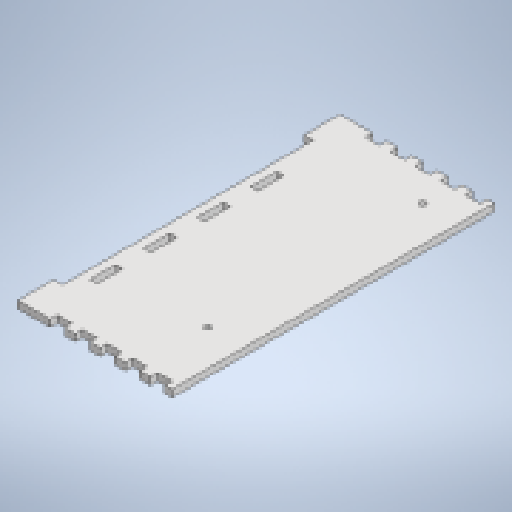
# Autodesk Inventor part: side
Saved by Autodesk Inventor 2025.3 (Build 293356000, 356)
## iProperties
Created: 2025-12-08
Part Number: side
Material: Generic
Document SubType Name: Modeling
Designer: hazem
Density: 1 g/cm^3
Appearance: Default
Author: hazem
Autodesk Inventor part; units mm, degrees
ref_plane "YZ Plane" through (0, 0, 0) normal (1, 0, 0) x (0, 1, 0)
ref_plane "XZ Plane" through (0, 0, 0) normal (0, 1, 0) x (-1, 0, 0)
ref_plane "XY Plane" through (0, 0, 0) normal (0, 0, 1) x (1, 0, 0)
sketch "Sketch1" plane through (0, 0, 0) normal (0, 1, 0) x (-1, 0, 0)
  line L0 (-9.6671, 163.8128) -> (70.4329, 163.8128)
  line L1 (70.4329, 163.8128) -> (70.4329, -16.1872)
  line L2 (70.4329, -16.1872) -> (-9.6671, -16.1872)
  line L3 (-9.6671, -16.1872) -> (-9.6671, 163.8128)
  point P0 (0, 0)
  constraints: 8 end point, 2 parallel, 1 horizontal, 1 perpendicular
extrude "Extrusion1" add sketch "Sketch1" along normal blind 4
sketch "Sketch2" plane through (0, 4, 0) normal (0, 1, 0) x (1, 0, 0)
  line L0 (-66.4329, -159.8128) -> (-66.4329, -148.8128) projected
  line L1 (-70.4329, -159.8128) -> (-70.4329, -148.8128) projected
  line L2 (-66.4329, -159.8128) -> (-66.4329, -148.8128) projected
  line L3 (-70.4329, -159.8128) -> (-70.4329, -148.8128) projected
  line L4 (-66.4329, -159.8128) -> (-66.4329, -148.8128) projected
  line L5 (-70.4329, -159.8128) -> (-70.4329, -148.8128) projected
  line L6 (-66.4329, -159.8128) -> (-66.4329, -148.8128) projected
  line L7 (-70.4329, -159.8128) -> (-70.4329, -148.8128) projected
  line L8 (-66.4329, -159.8128) -> (-66.4329, -148.8128) projected
  line L9 (-70.4329, -159.8128) -> (-70.4329, -148.8128) projected
  line L10 (-66.4329, -159.8128) -> (-66.4329, -148.8128) projected
  line L11 (-70.4329, -159.8128) -> (-70.4329, -148.8128) projected
  line L12 (-70.4329, -163.8128) -> (9.6671, -163.8128) projected
  line L13 (-30.3829, -163.8128) -> (-30.3829, 16.1872) construction
  line L14 (9.6671, 16.1872) -> (-70.4329, 16.1872) projected
  line L15 (-70.4329, -149.0628) -> (-66.4329, -149.0628)
  line L16 (-66.4329, -159.5628) -> (-70.4329, -159.5628)
  line L17 (-70.4329, 0.9372) -> (-66.4329, 0.9372)
  line L18 (-66.4329, -13.5628) -> (-70.4329, -13.5628)
  line L19 (-66.4329, -43.5628) -> (-70.4329, -43.5628)
  line L20 (-70.4329, -29.0628) -> (-66.4329, -29.0628)
  line L21 (-66.4329, -73.5628) -> (-70.4329, -73.5628)
  line L22 (-70.4329, -59.0628) -> (-66.4329, -59.0628)
  line L23 (-66.4329, -103.5628) -> (-70.4329, -103.5628)
  line L24 (-70.4329, -89.0628) -> (-66.4329, -89.0628)
  line L25 (-66.4329, -133.5628) -> (-70.4329, -133.5628)
  line L26 (-70.4329, -119.0628) -> (-66.4329, -119.0628)
  line L27 (5.6671, -159.8128) -> (5.6671, -148.8128)
  line L28 (9.6671, -159.8128) -> (9.6671, -148.8128)
  line L29 (5.6671, -133.8128) -> (5.6671, -118.8128)
  line L30 (9.6671, -133.8128) -> (9.6671, -118.8128)
  line L31 (5.6671, -103.8128) -> (5.6671, -88.8128)
  line L32 (9.6671, -103.8128) -> (9.6671, -88.8128)
  line L33 (5.6671, -73.8128) -> (5.6671, -58.8128)
  line L34 (9.6671, -73.8128) -> (9.6671, -58.8128)
  line L35 (5.6671, -43.8128) -> (5.6671, -28.8128)
  line L36 (9.6671, -43.8128) -> (9.6671, -28.8128)
  line L37 (5.6671, -13.8128) -> (5.6671, 1.1872)
  line L38 (9.6671, -13.8128) -> (9.6671, 1.1872)
  line L39 (9.6671, -149.0628) -> (5.6671, -149.0628)
  line L40 (5.6671, -159.5628) -> (9.6671, -159.5628)
  line L41 (9.6671, 0.9372) -> (5.6671, 0.9372)
  line L42 (5.6671, -13.5628) -> (9.6671, -13.5628)
  line L43 (5.6671, -43.5628) -> (9.6671, -43.5628)
  line L44 (9.6671, -29.0628) -> (5.6671, -29.0628)
  line L45 (5.6671, -73.5628) -> (9.6671, -73.5628)
  line L46 (9.6671, -59.0628) -> (5.6671, -59.0628)
  line L47 (5.6671, -103.5628) -> (9.6671, -103.5628)
  line L48 (9.6671, -89.0628) -> (5.6671, -89.0628)
  line L49 (5.6671, -133.5628) -> (9.6671, -133.5628)
  line L50 (9.6671, -119.0628) -> (5.6671, -119.0628)
  line L51 (-66.4329, -148.8128) -> (-70.4329, -148.8128) projected
  line L52 (-66.4329, -159.8128) -> (-70.4329, -159.8128) projected
  line L53 (-66.4329, -148.8128) -> (-70.4329, -148.8128) projected
  line L54 (-66.4329, -159.8128) -> (-70.4329, -159.8128) projected
  line L55 (-66.4329, -148.8128) -> (-70.4329, -148.8128) projected
  line L56 (-66.4329, -159.8128) -> (-70.4329, -159.8128) projected
  line L57 (-66.4329, -148.8128) -> (-70.4329, -148.8128) projected
  line L58 (-66.4329, -159.8128) -> (-70.4329, -159.8128) projected
  line L59 (-66.4329, -148.8128) -> (-70.4329, -148.8128) projected
  line L60 (-66.4329, -159.8128) -> (-70.4329, -159.8128) projected
  line L61 (-66.4329, -148.8128) -> (-70.4329, -148.8128) projected
  line L62 (-66.4329, -159.8128) -> (-70.4329, -159.8128) projected
  line L63 (-66.4329, -133.5628) -> (-66.4329, -119.0628)
  line L64 (-66.4329, -103.5628) -> (-66.4329, -89.0628)
  line L65 (-66.4329, -73.5628) -> (-66.4329, -59.0628)
  line L66 (-66.4329, -43.5628) -> (-66.4329, -29.0628)
  line L67 (-66.4329, -13.5628) -> (-66.4329, 0.9372)
  line L68 (-70.4329, 16.1872) -> (-70.4329, -163.8128) projected
  line L69 (9.6671, -163.8128) -> (9.6671, 16.1872) projected
  line L70 (1.6671, 16.1872) -> (1.6671, 12.1872)
  line L71 (1.6671, 12.1872) -> (-6.3329, 12.1872)
  line L72 (-6.3329, 12.1872) -> (-6.3329, 16.1872)
  line L73 (-12.3329, 16.1872) -> (-12.3329, 12.1872)
  line L74 (-12.3329, 12.1872) -> (-20.3329, 12.1872)
  line L75 (-20.3329, 12.1872) -> (-20.3329, 16.1872)
  line L76 (-26.3329, 16.1872) -> (-26.3329, 12.1872)
  line L77 (-26.3329, 12.1872) -> (-34.3329, 12.1872)
  line L78 (-34.3329, 12.1872) -> (-34.3329, 16.1872)
  line L79 (-40.3329, 16.1872) -> (-40.3329, 12.1872)
  line L80 (-40.3329, 12.1872) -> (-48.3329, 12.1872)
  line L81 (-48.3329, 12.1872) -> (-48.3329, 16.1872)
  line L82 (-54.3329, 16.1872) -> (-54.3329, 12.1872)
  line L83 (-54.3329, 12.1872) -> (-62.3329, 12.1872)
  line L84 (-62.3329, 12.1872) -> (-62.3329, 16.1872)
  line L85 (-12.3329, -73.8128) -> (-48.4329, -73.8128) construction
  line L86 (1.6671, -163.8128) -> (1.6671, -159.8128)
  line L87 (1.6671, -159.8128) -> (-6.3329, -159.8128)
  line L88 (-6.3329, -159.8128) -> (-6.3329, -163.8128)
  line L89 (-12.3329, -163.8128) -> (-12.3329, -159.8128)
  line L90 (-12.3329, -159.8128) -> (-20.3329, -159.8128)
  line L91 (-20.3329, -159.8128) -> (-20.3329, -163.8128)
  line L92 (-26.3329, -163.8128) -> (-26.3329, -159.8128)
  line L93 (-26.3329, -159.8128) -> (-34.3329, -159.8128)
  line L94 (-34.3329, -159.8128) -> (-34.3329, -163.8128)
  line L95 (-40.3329, -163.8128) -> (-40.3329, -159.8128)
  line L96 (-40.3329, -159.8128) -> (-48.3329, -159.8128)
  line L97 (-48.3329, -159.8128) -> (-48.3329, -163.8128)
  line L98 (-54.3329, -163.8128) -> (-54.3329, -159.8128)
  line L99 (-54.3329, -159.8128) -> (-62.3329, -159.8128)
  line L100 (-62.3329, -159.8128) -> (-62.3329, -163.8128)
  line L101 (9.6671, 1.1872) -> (5.6671, 1.1872)
  line L102 (9.6671, -13.8128) -> (5.6671, -13.8128)
  line L103 (9.6671, -28.8128) -> (5.6671, -28.8128)
  line L104 (9.6671, -43.8128) -> (5.6671, -43.8128)
  line L105 (9.6671, -58.8128) -> (5.6671, -58.8128)
  line L106 (5.6671, -73.8128) -> (9.6671, -73.8128)
  line L107 (9.6671, -88.8128) -> (5.6671, -88.8128)
  line L108 (9.6671, -103.8128) -> (5.6671, -103.8128)
  line L109 (9.6671, -118.8128) -> (5.6671, -118.8128)
  line L110 (9.6671, -133.8128) -> (5.6671, -133.8128)
  line L111 (9.6671, -148.8128) -> (5.6671, -148.8128)
  line L112 (9.6671, -159.8128) -> (5.6671, -159.8128)
  circle A0 centre (-14.3329, -3.8128) radius 1.75
  circle A1 centre (-14.3329, -123.8128) radius 1.75
  line L113 (5.6671, -163.8128) -> (5.6671, 16.1872)
  point P0 (0, 0)
  point P1 (-30.3829, -73.8128)
  point P2 (5.6671, 1.1872)
  dimension "d6" = 30
  dimension "d13" = 4
  dimension "d14" = 8
  dimension "d15" = 4
  dimension "d16" = 8
  dimension "d19" = 14
  dimension "d24" = 180
  dimension "d30" = 3.5
  dimension "d31" = 40
  dimension "d32" = 20
  dimension "d33" = 24
  constraints: 172 end point, 48 symmetric about line, 21 point on line, 12 parallel, 4 collinear, 4 midpoint, 3 horizontal, 3 vertical, 2 centre point, 1 equal radius, 1 perpendicular, 1 vertical alignment, 54 other
  measures "d6" distance of L18.start L19.start
  measures "d13" distance of L70.start L70.end
  measures "d14" distance of L70.end L71.end
  measures "d15" distance of L71.end L72.end
  measures "d19" distance of L70.start L73.start
  measures "d24" distance between parallel lines of L12 L14
  measures "d30" diameter of A1
  measures "d31" distance from line of L12 A1.centre
  measures "d32" distance from line of L14 A0.centre
extrude "Extrusion2" cut sketch "Sketch2" against normal up to surface (4 mm away) contours L16 L1 L15 L0 | L100 L99 L98 L12 | L68 L26 L63 L25 | L97 L96 L95 L12 | L68 L24 L64 L23 | L94 L93 L92 L12 | L68 L22 L65 L21 | L91 L90 L89 L12 | L68 L20 L66 L19 | L88 L87 L86 L12 | L68 L17 L67 L18 | L113 L112 L69 L12 | L27 L40 L28 L112 | L27 L39 L28 L40 | L14 L82 L83 L84 | L27 L111 L28 L39 | L113 L110 L69 L111 | L14 L79 L80 L81 | L29 L49 L30 L110 | L29 L50 L30 L49 | L14 L76 L77 L78 | L29 L109 L30 L50 | L113 L108 L69 L109 | L14 L73 L74 L75 | L31 L47 L32 L108 | L31 L48 L32 L47 | L14 L70 L71 L72 | L31 L107 L32 L48 | L113 L106 L69 L107 | L14 L69 L101 L113 | L33 L45 L34 L106 | L101 L38 L41 L37 | L33 L46 L34 L45 | L41 L38 L42 L37 | L33 L105 L34 L46 | L42 L38 L102 L37 | L113 L104 L69 L105 | L102 L69 L103 L113 | L35 L43 L36 L104 | L103 L36 L44 L35 | L35 L44 L36 L43 | A0 | A1
sketch "Sketch4" plane through (0, 0, 0) normal (0, -1, 0) x (1, 0, 0)
  line L0 (-66.4329, 149.0628) -> (-70.4329, 149.0628) projected
  line L1 (-70.4329, 159.5628) -> (-70.4329, 163.8128) projected
  line L2 (-66.4329, 149.0628) -> (-70.4329, 149.0628)
  line L3 (-70.4329, 143.8128) -> (-70.4329, 159.5628)
  line L4 (-70.4329, 159.5628) -> (-66.4329, 159.5628)
  line L5 (-66.4329, 159.5628) -> (-66.4329, 149.0628)
  line L6 (-70.4329, 163.8128) -> (-80.4329, 163.8128)
  line L7 (-80.4329, 163.8128) -> (-80.4329, 143.8128)
  line L8 (-80.4329, 143.8128) -> (-70.4329, 143.8128)
  line L9 (-70.4329, 143.8128) -> (-70.4329, 163.8128)
  line L10 (-70.4329, -16.1872) -> (-70.4329, -0.9372) projected
  line L11 (-66.4329, 13.5628) -> (-70.4329, 13.5628)
  line L12 (-70.4329, 133.5628) -> (-70.4329, -0.9372)
  line L13 (-70.4329, -0.9372) -> (-66.4329, -0.9372)
  line L14 (-66.4329, -0.9372) -> (-66.4329, 13.5628)
  line L15 (-70.4329, 13.5628) -> (-66.4329, 13.5628) projected
  line L16 (-70.4329, -16.1872) -> (-80.4329, -16.1872)
  line L17 (-80.4329, -16.1872) -> (-80.4329, 3.8128)
  line L18 (-80.4329, 3.8128) -> (-70.4329, 3.8128)
  line L19 (-70.4329, 3.8128) -> (-70.4329, -16.1872)
  line L20 (-75.4329, 143.8128) -> (-75.4329, 3.8128)
  line L21 (-40.3329, 163.8128) -> (-40.3329, 159.8128) projected
  line L22 (-40.3329, 159.8128) -> (-48.3329, 159.8128) projected
  line L23 (-48.3329, 159.8128) -> (-48.3329, 163.8128) projected
  line L24 (-54.3329, 163.8128) -> (-48.3329, 163.8128) projected
  line L25 (-54.3329, 163.8128) -> (-54.3329, 159.8128) projected
  line L26 (-54.3329, 159.8128) -> (-62.3329, 159.8128) projected
  line L27 (-62.3329, 159.8128) -> (-62.3329, 163.8128) projected
  line L28 (-70.4329, 163.8128) -> (-62.3329, 163.8128) projected
  line L29 (-70.4329, 159.5628) -> (-70.4329, 163.8128) projected
  line L30 (-70.4329, 159.5628) -> (-66.4329, 159.5628) projected
  line L31 (-66.4329, 159.5628) -> (-66.4329, 149.0628) projected
  line L32 (-66.4329, 149.0628) -> (-70.4329, 149.0628) projected
  line L33 (-70.4329, 133.5628) -> (-70.4329, 149.0628) projected
  line L34 (-70.4329, 133.5628) -> (-66.4329, 133.5628) projected
  line L35 (-66.4329, 133.5628) -> (-66.4329, 119.0628) projected
  line L36 (-66.4329, 119.0628) -> (-70.4329, 119.0628) projected
  line L37 (-70.4329, 103.5628) -> (-70.4329, 119.0628) projected
  line L38 (-70.4329, 103.5628) -> (-66.4329, 103.5628) projected
  line L39 (-66.4329, 103.5628) -> (-66.4329, 89.0628) projected
  line L40 (-66.4329, 89.0628) -> (-70.4329, 89.0628) projected
  line L41 (-70.4329, 73.5628) -> (-70.4329, 89.0628) projected
  line L42 (-70.4329, 73.5628) -> (-66.4329, 73.5628) projected
  line L43 (-66.4329, 73.5628) -> (-66.4329, 59.0628) projected
  line L44 (-66.4329, 59.0628) -> (-70.4329, 59.0628) projected
  line L45 (-70.4329, 43.5628) -> (-70.4329, 59.0628) projected
  line L46 (-70.4329, 43.5628) -> (-66.4329, 43.5628) projected
  line L47 (-66.4329, 43.5628) -> (-66.4329, 29.0628) projected
  line L48 (-66.4329, 29.0628) -> (-70.4329, 29.0628) projected
  line L49 (-70.4329, 13.5628) -> (-70.4329, 29.0628) projected
  line L50 (-70.4329, 13.5628) -> (-66.4329, 13.5628) projected
  line L51 (-66.4329, 13.5628) -> (-66.4329, -0.9372) projected
  line L52 (-66.4329, -0.9372) -> (-70.4329, -0.9372) projected
  line L53 (-70.4329, -16.1872) -> (-70.4329, -0.9372) projected
  line L54 (-62.3329, -16.1872) -> (-70.4329, -16.1872) projected
  line L55 (-62.3329, -16.1872) -> (-62.3329, -12.1872) projected
  line L56 (-62.3329, -12.1872) -> (-54.3329, -12.1872) projected
  line L57 (-54.3329, -12.1872) -> (-54.3329, -16.1872) projected
  line L58 (-48.3329, -16.1872) -> (-54.3329, -16.1872) projected
  line L59 (-48.3329, -16.1872) -> (-48.3329, -12.1872) projected
  line L60 (-48.3329, -12.1872) -> (-40.3329, -12.1872) projected
  line L61 (-40.3329, -12.1872) -> (-40.3329, -16.1872) projected
  line L62 (-34.3329, -16.1872) -> (-40.3329, -16.1872) projected
  line L63 (-34.3329, -16.1872) -> (-34.3329, -12.1872) projected
  line L64 (-34.3329, -12.1872) -> (-26.3329, -12.1872) projected
  line L65 (-26.3329, -12.1872) -> (-26.3329, -16.1872) projected
  line L66 (-20.3329, -16.1872) -> (-26.3329, -16.1872) projected
  line L67 (-20.3329, -16.1872) -> (-20.3329, -12.1872) projected
  line L68 (-20.3329, -12.1872) -> (-12.3329, -12.1872) projected
  line L69 (-12.3329, -12.1872) -> (-12.3329, -16.1872) projected
  line L70 (-6.3329, -16.1872) -> (-12.3329, -16.1872) projected
  line L71 (-6.3329, -16.1872) -> (-6.3329, -12.1872) projected
  line L72 (-6.3329, -12.1872) -> (1.6671, -12.1872) projected
  line L73 (1.6671, -12.1872) -> (1.6671, -16.1872) projected
  line L74 (5.6671, -16.1872) -> (1.6671, -16.1872) projected
  line L75 (1.6671, 163.8128) -> (5.6671, 163.8128) projected
  line L76 (1.6671, 163.8128) -> (1.6671, 159.8128) projected
  line L77 (1.6671, 159.8128) -> (-6.3329, 159.8128) projected
  line L78 (-6.3329, 159.8128) -> (-6.3329, 163.8128) projected
  line L79 (-12.3329, 163.8128) -> (-6.3329, 163.8128) projected
  line L80 (-12.3329, 163.8128) -> (-12.3329, 159.8128) projected
  line L81 (-12.3329, 159.8128) -> (-20.3329, 159.8128) projected
  line L82 (-20.3329, 159.8128) -> (-20.3329, 163.8128) projected
  line L83 (-26.3329, 163.8128) -> (-20.3329, 163.8128) projected
  line L84 (-26.3329, 163.8128) -> (-26.3329, 159.8128) projected
  line L85 (-26.3329, 159.8128) -> (-34.3329, 159.8128) projected
  line L86 (-34.3329, 159.8128) -> (-34.3329, 163.8128) projected
  line L87 (-40.3329, 163.8128) -> (-34.3329, 163.8128) projected
  line L88 (5.6671, -16.1872) -> (5.6671, 163.8128) projected
  point P0 (0, 0)
  dimension "d25" = 10
  dimension "d26" = 20
  dimension "d29" = 5
  constraints: 34 end point, 8 parallel, 5 perpendicular, 4 horizontal, 4 point on line, 2 equal length, 2 midpoint, 1 collinear
  measures "d25" distance of L3.start L7.end
  measures "d26" distance of L7.end L6.end
  measures "d29" distance between parallel lines of L12 L20
extrude "Extrusion3" add sketch "Sketch4" against normal up to surface (4 mm away) contours L0 L3 L4 L5 | L3 L8 L7 L6 L1 | L33 L12 L18 L20 L8 | L18 L12 L10 L16 L17 | L12 L11 L14 L13
body "Solid1"
